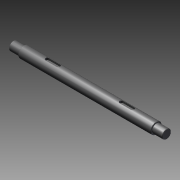
# Autodesk Inventor part: NSFRQ15-181-F14-P12-T14-Q12-WKC30-C20-K30-E20_s
Saved by Autodesk Inventor 2011 SP1 (Build 150282100, 282)
## iProperties
Created: 2016-11-24
Part Number: NSFRQ15-181-F14-P12-T14-Q12-WKC30-C20-K30-E20_s
Catalog Web Link: www.cadenas.de
Description: NSFRMHQ, SFRMHQ, PSFRMHQ, SSFRMHQ, NSFRMGQ, SFRMGQ, PSFRMGQ, SSFRMGQ, NSFRHQ, SFRHQ, PSFRHQ, SSFRHQ, NSFRQ, SFRQ, PSFRQ, SSFRQ, HFRQ, PHFRQ_shaft-Rotary Shafts - Both Ends Stepped -
Vendor: MISUMI
Document SubType Name: Modeling
Designer: psAdmin
Manufacturer: MISUMI
Mass: 34.5896 g
Surface Area: 101.193 cm^2
Volume: 34.5896 cm^3
Density: 1 g/cm^3
Category: PARTsolutions
Company: MISUMI
Title: NSFRQ15-181-F14-P12-T14-Q12-WKC30-C20-K30-E20
Author: Cadenas PARTsolutions
Comments: Rotary Shafts - Both Ends Stepped -
PSOL_IDENT_0: {$CADENAS_DATA\23d-libs\misumi\metric\11_rotary_shafts\11_components\phfrq\phfrq.prj},671 {VTYP=3D},
PSOL_IDENT_1: {NB=NSFRQ15-181-F14-P12-T14-Q12-WKC30-C20-K30-E20_s},{LINA=NSFRQ15-181-F14-P12-T14-Q12-WKC30-C20-K30
PSOL_IDENT_2: -E20},{NN=NSFRMHQ, SFRMHQ, PSFRMHQ, SSFRMHQ, NSFRMGQ, SFRMGQ, PSFRMGQ, SSFRMGQ, NSFRHQ, SFRHQ, PSFRH
PSOL_IDENT_3: Q, SSFRHQ, NSFRQ, SFRQ, PSFRQ, SSFRQ, HFRQ, PHFRQ_shaft},{DATE=20.09.2016 01:43:22},{GEOMDATE=16.09.
PSOL_IDENT_4: 2016 05:13:09},{VERSION=},{LINEID=70},{LINESUBID=-1},{WBVAR=TS,TYS,MAT,ST,ALT1,L,ALT9,F,P,T,Q,ALT2,K
PSOL_IDENT_5: C,A,WKC,C,K,E,KZ,Z,ALT8,PKC,ALT14,QKC,ALT21,PP,PK,ALT22,QQ,QK,ALT23,PV,PW,ALT24,QV,QW,ALT27,TL,TR,AL
PSOL_IDENT_6: T28,TF,ALT29,TTALT29,ALT3,FC,GALT3,WFC,J,WALT3,V,ALT4,SFC,SG,AG,ALT25,PFC,LC,ALT26,QFC,RC,ALT10,KWC,
PSOL_IDENT_7: ALT11,WC,ALT5,UC,ALT7,SC,ALT33,CPALT33,CQALT33,ALT30,PM,QM}  {NB=NSFRQ15-181-F14-P12-T14-Q12-WKC30-C
PSOL_IDENT_8: 20-K30-E20_s},{LINA=NSFRQ15-181-F14-P12-T14-Q12-WKC30-C20-K30-E20},{KT=DUMMY},{PN=NSFRQ15-181-F14-P1
PSOL_IDENT_9: 2-T14-Q12-WKC30-C20-K30-E20},{TYPE=NSFRQ},{TS=},{TYS=},{TYSALG='','g6'},{TYSS=},{TSALG='M','h9 (Cold
PSOL_IDENT_10: -drawn)','H','h7 (Ground)','','g6 (Ground)'},{MAT=S45C},{MATALG= 'S45C','S45C Equivalent', 'SUS304','
PSOL_IDENT_11: SUS304', 'SCM435','4137 Alloy Steel' },{ST=},{STALG= '','-','BO','Black Oxide', 'ENP','Electroless N
PSOL_IDENT_12: ickel Plating' },{D=15},{ALT1=},{L=181.0},{LALG=[15:796/0.1]},{LMIN=15},{LMAX=796},{LMAXLKC=799.9},{
PSOL_IDENT_13: ALT9=},{ALT9ALG= '', 'w/o CKC (Concentricity)','-CKC', 'with CKC (Concentricity)' },{F=14.0},{FALG=[
PSOL_IDENT_14: 2:70/0.1]},{FMIN=2},{FMAX=70},{P=12},{PALG=[5:14/1]},{PMIN=5},{PMIN2=0},{PMAX=14},{T=14.0},{TALG=[2:
PSOL_IDENT_15: 70/0.1]},{TMIN=2},{TMAX=70},{Q=12},{QALG=[5:14/1]},{QMIN=5},{QMIN2=0},{QMAX=14},{CIFC=0},{CC=0.5},{C
PSOL_IDENT_16: C1=0.5},{Y=800},{ALT2=WKC},{ALT2ALG= '', 'w/o Key Grooves','KC','with KC (Key Groove)','WKC','with W
PSOL_IDENT_17: KC (Two Key Grooves)','KCWKC','with KC + WKC (Three Key Grooves)','KZ','with KC + WKC + KZ (Four Key
PSOL_IDENT_18: Grooves)' },{ALT2PN=-WKC30-C20-K30-E20},{KC=0.0},{KCALG=[0]},{KCMIN=0},{KCMAX=176},{KCMAX2=166},{KC
PSOL_IDENT_19: MAX3=161},{A=0.0},{AALG=[0]},{AMIN=5},{AMAX=100},{AMAX2=100},{AMAX3=100},{WKC=30.0},{WKCALG=[0:171/0
PSOL_IDENT_20: .1]},{WKCMIN=0},{WKCMIN2=0},{WKCMAX=171},{WKCMAX2=166},{C=20.0},{CALG=[5:100/0.1]},{CMIN=5},{CMAX=10
PSOL_IDENT_21: 0},{CMAX2=100},{K=30.0},{KALG=[0:126/0.1]},{KMIN=0},{KMIN2=5},{KMAX=126},{E=20.0},{EALG=[5:100/0.1]}
PSOL_IDENT_22: ,{EMIN=5},{EMAX=100},{KZ=0.0},{KZALG=[0]},{KZMIN=151},{KZMAX=176},{Z=0.0},{ZALG=[0]},{ZMIN=5},{ZMAX=
PSOL_IDENT_23: 100},{BBALT2=5},{TTALT2=3},{ALT8=},{ALT8ALG= '','w/o PKC (Keyway on Step P (Position Zero from End F
PSOL_IDENT_24: ace))','PKC','with PKC (Keyway on Step P (Position Zero from End Face))' },{ALT8PN=},{PKC=0.0},{PKCA
PSOL_IDENT_25: LG=[0]},{PKCMIN=4},{PKCMAX=14},{ALT14=},{ALT14ALG= '','w/o QKC (Keyway on Step Q (Position Zero from
PSOL_IDENT_26: End Face))','QKC','with QKC (Keyway on Step Q (Position Zero from End Face))' },{ALT14PN=},{QKC=0.0
PSOL_IDENT_27: },{QKCALG=[0]},{QKCMIN=4},{QKCMAX=14},{ALT21=},{ALT21ALG= '','w/o PP (Keyway on Step P (Position Spe
PSOL_IDENT_28: cfied))','PP','with PP (Keyway on Step P (Position Specfied))' },{ALT21PN=},{BBALT21=2},{PP=0.0},{PP
PSOL_IDENT_29: ALG=[0]},{PPMIN1=0},{PPMIN2=0},{PPMAX=10},{PK=0.0},{PKALG=[0]},{PKMIN=4},{PKMAX=14},{ALT22=},{ALT22A
PSOL_IDENT_30: LG= '','w/o QQ (Keyway on Step Q (Position Specfied))','QQ','with QQ (Keyway on Step Q (Position Spe
PSOL_IDENT_31: cfied))' },{ALT22PN=},{QQ=0.0},{QQALG=[0]},{QQMIN1=0},{QQMIN2=0},{QQMAX=10},{QK=0.0},{QKALG=[0]},{QK
PSOL_IDENT_32: MIN=4},{QKMAX=14},{ALT23=},{ALT23ALG= '','Not applicable' },{ALT23PN=},{PV=0.0},{PVALG=[0]},{PVMIN=0
PSOL_IDENT_33: },{PVMAX=10},{PW=0.0},{PWALG=[0]},{PWMIN=4},{PWMAX=14},{ALT24=},{ALT24ALG= '','Not applicable' },{AL
PSOL_IDENT_34: T24PN=},{QV=0.0},{QVALG=[0]},{QVMIN=0},{QVMAX=10},{QW=0.0},{QWALG=[0]},{QWMIN=4},{QWMAX=14},{ALT27=}
PSOL_IDENT_35: ,{ALT27ALG= '','w/o Retaining Ring Groove at D','TL','with TL (Retaining Ring Groove at D)','TR','wi
PSOL_IDENT_36: th TR (Retaining Ring Groove at D)','TLTR','with TL + TR (Retaining Ring Groove at D)' },{ALT27PN=},
PSOL_IDENT_37: {TL=0.0},{TLALG=[0]},{TLMIN=3.2},{TLMAX=0},{TR=0.0},{TRALG=[0]},{TRMIN=3.2},{TRMAX=0},{MMALT27=1.15}
PSOL_IDENT_38: ,{DDDALT27=0},{ALT28=},{ALT28ALG= '','w/o TF (Retaining Ring Groove at Step P)','TF','with TF (Retai
PSOL_IDENT_39: ning Ring Groove at Step P)' },{ALT28PN=},{TF=0.0},{TFALG=[0]},{TFMIN=3.2},{TFMAX=12},{MMALT28ALG=1.
PSOL_IDENT_40: 15},{MMALT28=0},{DDDALT28=0},{ALT29=},{ALT29ALG= '','w/o TT (Retaining Ring Groove at Step Q)','TT','
PSOL_IDENT_41: with TT (Retaining Ring Groove at Step Q)' },{ALT29PN=},{TTALT29=0.0},{TTALT29ALG=[0]},{TTALT29MIN=3
PSOL_IDENT_42: .2},{TTALT29MAX=12},{MMALT29=0},{MMALT29ALG=1.15},{DDDALT29=0},{ALT3=},{ALT3ALG= '', 'w/o Set Screw
PSOL_IDENT_43: Flat','FC','with FC (Adds a Set Screw Flat)','WFC','with WFC (Adds Two Set Screw Flats)','FCWFC','wi
PSOL_IDENT_44: th FC + WFC (Adds Three Set Screw Flats)' },{ALT3PN=},{FC=0},{FCALG=[0]},{FCMIN=0},{FCMAX=180},{GALT
PSOL_IDENT_45: 3=0},{GALT3ALG=[0]},{GALT3MIN=1},{GALT3MAX=70},{GALT3MAX2=70},{GALT3MAX3=70},{WFC=0},{WFCALG=[0]},{W
PSOL_IDENT_46: FCMIN=0},{WFCMIN2=2},{WFCMAX=177},{WFCMAX2=-3},{WFCMAX3=-4},{J=0},{JALG=[0]},{JMIN=1},{JMAX=70},{JMA
PSOL_IDENT_47: X2=-2},{JMAX3=-5},{WALT3=0},{WALT3ALG=[0]},{WALT3MIN=0},{WALT3MIN2=183},{WALT3MAX=178},{WALT3MAX2=17
PSOL_IDENT_48: 8},{V=0},{VALG=[0]},{VMIN=1},{VMAX=70},{VMAX2=70},{CIFCUT=0},{CIFFC=0},{ALT4=},{ALT4ALG= '', 'w/o SF
PSOL_IDENT_49: C (2 Set Screw Flats (Angle Specified))', 'SFC' , 'with SFC (2 Set Screw Flats (Angle Specified))'},
PSOL_IDENT_50: {ALT4PN=},{SFC=0},{SFCALG=[0]},{SFCMIN=0},{SFCMAX=180},{SG=0},{SGALG=[0]},{SGMIN=1},{SGMAX=70},{AG=0
PSOL_IDENT_51: },{AGALG=[0]},{HALT4=0},{CIFSFC=0},{CUTSFC=0},{ALT25=},{ALT25ALG= '','w/o PFC (Set Screw Flat on Ste
PSOL_IDENT_52: p P)','PFC','with PFC (Set Screw Flat on Step P)' },{ALT25PN=},{PFC=0},{PFCALG=[0]},{PFCMN=0},{PFCMA
PSOL_IDENT_53: X=13},{LC=0},{LCALG=[0]},{LCMIN=1},{LCMAX=14},{HALT25=0},{ALT26ALG= '','w/o QFC (Set Screw Flat on S
PSOL_IDENT_54: tep Q)','QFC','with QFC (Set Screw Flat on Step Q)' },{ALT26=},{ALT26PN=},{QFC=0},{QFCALG=[0]},{QFCM
PSOL_IDENT_55: IN=0},{QFCMAX=13},{RC=0},{RCALG=[0]},{RCMIN=1},{RCMAX=14},{HALT26=0},{ALT10=},{ALT10ALG= '','w/o KWC
PSOL_IDENT_56: (2 Set Screw Flats at both ends)','KWC','with KWC (2 Set Screw Flats at both ends)' },{ALT10PN=},{K
PSOL_IDENT_57: WC=0},{KWCALG=0},{HALT10P=1.0},{HALT10Q=1.0},{ALT11=},{ALT11ALG= '','Not applicable' },{ALT11PN=},{W
PSOL_IDENT_58: C=0.0},{WCALG=0},{WCMAX=11.9},{WC1=10},{WC1MIN=9.9},{WC1MAX=10.1},{ALT5=},{ALT5ALG= '','Not applicab
PSOL_IDENT_59: le' },{ALT5PN=},{UC=0},{UCALG=[0]},{UCMIN=1},{UCMAX=175},{DD=0},{LL1=0},{ALT7=},{ALT7ALG= '', 'w/o S
PSOL_IDENT_60: C (Wrench Flats)', 'SC', 'with SC (Wrench Flats)'},{ALT7PN=},{SC=0},{SCALG=[0]},{SCMIN=0},{SCMAX=171
PSOL_IDENT_61: },{WALT7=0},{LL2=0},{LL2ALG=10},{CIFSC=0},{CUTSC=0},{TPKC=0.2},{BBALT8=4},{TTALT8=2.5},{CIFPKC=0},{T
PSOL_IDENT_62: QKC=0.2},{BBALT14=4},{TTALT14=2.5},{CIFQKC=0},{CIFR=0},{CIFR2=0},{ERRORPN=},{ERRORALT23=OK},{ERRORAL
PSOL_IDENT_63: T24=OK},{ERRORALT25=OK},{ERRORALT27=OK},{ERRORALT28=OK},{ERRORALT210=OK},{ERRORALT214=OK},{ERRORALT3
PSOL_IDENT_64: 4=OK},{ERRORALT35=OK},{ERRORALT37=OK},{ERRORALT45=OK},{ERRORALT47=OK},{ERRORALT57=OK},{CIFKG=2},{KGM
PSOL_IDENT_65: IN1=30},{KGMAX1=50},{KGMIN2=131},{KGMAX2=151},{KGMIN3=0},{KGMAX3=0},{KGMIN4=0},{KGMAX4=0},{CIFKGC=2}
PSOL_IDENT_66: ,{CIFKG1=0},{CIFKG2=0},{CIFKG3=0},{CIFKG4=0},{CIFKGPCUT=0},{CIFKGQCUT=0},{PCUT3D=0},{QCUT3D=0},{CIFK
PSOL_IDENT_67: GP=0},{KGPMIN1=0},{KGPMAX1=0},{KGPMIN2=0},{KGPMAX2=0},{KGPMIN3=0},{KGPMAX3=0},{CIFKGPC=0},{CIFKGP1=1
PSOL_IDENT_68: },{CIFKGQ=0},{KGQMIN1=0},{KGQMAX1=0},{KGQMIN2=0},{KGQMAX2=0},{KGQMIN3=0},{KGQMAX3=0},{CIFKGQC=0},{CI
PSOL_IDENT_69: FKGQ1=1},{ALT33=},{ALT33ALG= '', 'w/o Step Chamfering','CP','with CP (Step P Chamfering)','CQ','with
PSOL_IDENT_70: CQ (Step Q Chamfering)','CPCQ','with CP + CQ (Step Chamfering at Both Steps)' },{ALT33PN=},{CPALT33=
PSOL_IDENT_71: },{CPALT33ALG= '','N/A' },{CPALT333D=0.5},{CQALT33=},{CQALT33ALG= '','N/A' },{CQALT333D=0.5},{CIF33P
PSOL_IDENT_72: FC=0},{CIF33QFC=0},{CIF33KWCP=0},{CIF33KWCQ=0},{CIF33TFP=0},{CIF33TTQ=0},{ERRORALT221=OK},{ERRORALT2
PSOL_IDENT_73: 22=OK},{ERRORALT223=OK},{ERRORALT224=OK},{ERRORALT225=OK},{ERRORALT226=OK},{ERRORALT227=OK},{ERRORAL
PSOL_IDENT_74: T228=OK},{ERRORALT229=OK},{ERRORALT230=OK},{ERRORALT310=OK},{ERRORALT327=OK},{ERRORALT330=OK},{ERROR
PSOL_IDENT_75: ALT410=OK},{ERRORALT427=OK},{ERRORALT430=OK},{ERRORALT510=OK},{ERRORALT527=OK},{ERRORALT530=OK},{ERR
PSOL_IDENT_76: ORALT710=OK},{ERRORALT730=OK},{ERRORALT825=OK},{ERRORALT828=OK},{ERRORALT830=OK},{ERRORALT1030=OK},{
PSOL_IDENT_77: ERRORALT1426=OK},{ERRORALT1429=OK},{ERRORALT1430=OK},{ERRORALT2125=OK},{ERRORALT2128=OK},{ERRORALT21
PSOL_IDENT_78: 30=OK},{ERRORALT2226=OK},{ERRORALT2229=OK},{ERRORALT2230=OK},{ERRORALT2325=OK},{ERRORALT2328=OK},{ER
PSOL_IDENT_79: RORALT2426=OK},{ERRORALT2429=OK},{ERRORALT2528=OK},{ERRORALT2530=OK},{ERRORALT2629=OK},{ERRORALT2630=
PSOL_IDENT_80: OK},{ERRORALT2830=OK},{ERRORALT2930=OK},{ALT30=},{ALT30ALG= '','w/o Tapping','PM','with PM (Tapping)'
PSOL_IDENT_81: ,'QM','with QM (Tapping)','PMQM','with PM + QM (Tapping)' },{ALT30PN=},{PM=0},{PMALG= 0 },{QM=0},{QM
PSOL_IDENT_82: ALG=0},{PM3D=0},{QM3D=0},{CIFPM=0},{CIFQM=0},{PMPITCH=0},{QMPITCH=0},{PMDEEP=0},{QMDEEP=0},{CIFCALC1=
PSOL_IDENT_83: 20},{CIFCALC2=20},{CIFCALC3=0},{CIFCALC4=0},{CIFPCALC1=0},{CIFPCALC2=0},{CIFPCALC3=0},{CIFQCALC1=0},
PSOL_IDENT_84: {CIFQCALC2=0},{CIFQCALC3=0},{QMALG1=0},{QMALG2=0}
NN: NSFRMHQ, SFRMHQ, PSFRMHQ, SSFRMHQ, NSFRMGQ, SFRMGQ, PSFRMGQ, SSFRMGQ, NSFRHQ, SFRHQ, PSFRHQ, SSFRHQ, NSFRQ, SFRQ, PSFRQ, SSFRQ, HFRQ, PHFRQ_shaft
NT: Rotary Shafts - Both Ends Stepped -
NB: NSFRQ15-181-F14-P12-T14-Q12-WKC30-C20-K30-E20_s
NBSYN: $PN._s
LINA: NSFRQ15-181-F14-P12-T14-Q12-WKC30-C20-K30-E20
PN: NSFRQ15-181-F14-P12-T14-Q12-WKC30-C20-K30-E20
TS: g6 (Ground)
TYS: g6
MAT: S45C Equivalent
ST: -
D: 15
ALT1: w/o LKC (Changes L Tolerance)
L: 181.0
ALT9: w/o CKC (Concentricity)
F: 14.0
P: 12
T: 14.0
Q: 12
Y: 800
ALT2: with WKC (Two Key Grooves)
KC: 0.0
A: 0.0
WKC: 30.0
C: 20.0
K: 30.0
E: 20.0
KZ: 0.0
Z: 0.0
ALT8: w/o PKC (Keyway on Step P (Position Zero from End Face))
PKC: 0.0
ALT14: w/o QKC (Keyway on Step Q (Position Zero from End Face))
QKC: 0.0
ALT21: w/o PP (Keyway on Step P (Position Specfied))
PP: 0.0
PK: 0.0
ALT22: w/o QQ (Keyway on Step Q (Position Specfied))
QQ: 0.0
QK: 0.0
ALT23: Not applicable
PV: 0.0
PW: 0.0
ALT24: Not applicable
QV: 0.0
QW: 0.0
ALT27: w/o Retaining Ring Groove at D
TL: 0.0
TR: 0.0
ALT28: w/o TF (Retaining Ring Groove at Step P)
TF: 0.0
ALT29: w/o TT (Retaining Ring Groove at Step Q)
TTALT29: 0.0
ALT3: w/o Set Screw Flat
FC: 0
GALT3: 0
WFC: 0
J: 0
WALT3: 0
V: 0
ALT4: w/o SFC (2 Set Screw Flats (Angle Specified))
SFC: 0
SG: 0
AG: 0
HALT4: 0
ALT25: w/o PFC (Set Screw Flat on Step P)
PFC: 0
LC: 0
ALT26: w/o QFC (Set Screw Flat on Step Q)
QFC: 0
RC: 0
ALT10: w/o KWC (2 Set Screw Flats at both ends)
KWC: 0
ALT11: Not applicable
WC: 0.0
ALT5: Not applicable
UC: 0
DD: 0
LL1: 0
ALT7: w/o SC (Wrench Flats)
SC: 0
WALT7: 0
LL2: 0
ALT33: w/o Step Chamfering
CPALT33: N/A
CQALT33: N/A
ALT30: w/o Tapping
PM: 0
QM: 0
SUPPLIER: MISUMI
ARTICLENO: NSFRQ15-181-F14-P12-T14-Q12-WKC30-C20-K30-E20_s
BOMINFO: NSFRQ15-181-F14-P12-T14-Q12-WKC30-C20-K30-E20
CREATOR: CADENAS GmbH
Autodesk Inventor part; units mm, degrees
ref_plane "YZ Plane" through (0, 0, 0) normal (1, 0, 0) x (0, 1, 0)
ref_plane "XZ Plane" through (0, 0, 0) normal (0, 1, 0) x (-1, 0, 0)
ref_plane "XY Plane" through (0, 0, 0) normal (0, 0, 1) x (1, 0, 0)
sketch "Sketch_1" plane through (0, 0, 0) normal (0, 0, 1) x (1, 0, 0)
  line L0 (195, 0) -> (-14, 0)
  line L1 (-14, 0) -> (-14, 5.5)
  line L2 (-14, 5.5) -> (-13.5, 6)
  line L3 (-13.5, 6) -> (-0.2, 6)
  arc A0 (-0.2, 6) -> (0, 6.2) centre (-0.2, 6.2) ccw
  line L4 (0, 6.2) -> (0, 7)
  line L5 (0, 7) -> (0.5, 7.5)
  line L6 (0.5, 7.5) -> (180.5, 7.5)
  line L7 (180.5, 7.5) -> (181, 7)
  line L8 (181, 7) -> (181, 6.2)
  arc A1 (181, 6.2) -> (181.2, 6) centre (181.2, 6.2) ccw
  line L9 (181.2, 6) -> (194.5, 6)
  line L10 (194.5, 6) -> (195, 5.5)
  line L11 (195, 5.5) -> (195, 0)
  line L12 (195, 0) -> (-14, 0)
  constraints: 26 end point, 4 point on circle, 2 centre point
revolve "Revolution1" add sketch "Sketch_1" angle 360 about axis through (195, 0, 0) along (1, 0, 0)
sketch "_____2" plane through (0, 0, 7.5) normal (0, 0, 1) x (1, 0, 0)
  arc A0 (32.5, 2.5) -> (32.5, -2.5) centre (32.5, 0) ccw
  line L0 (32.5, -2.5) -> (47.5, -2.5)
  arc A1 (47.5, -2.5) -> (47.5, 2.5) centre (47.5, 0) ccw
  line L1 (47.5, 2.5) -> (32.5, 2.5)
  constraints: 4 end point, 4 point on circle, 2 centre point
extrude "Extrusion1" cut sketch "_____2" against normal blind 3
sketch "_____6" plane through (0, 0, 7.5) normal (0, 0, 1) x (1, 0, 0)
  arc A0 (133.5, 2.5) -> (133.5, -2.5) centre (133.5, 0) ccw
  line L0 (133.5, -2.5) -> (148.5, -2.5)
  arc A1 (148.5, -2.5) -> (148.5, 2.5) centre (148.5, 0) ccw
  line L1 (148.5, 2.5) -> (133.5, 2.5)
  constraints: 4 end point, 4 point on circle, 2 centre point
extrude "Extrusion2" cut sketch "_____6" against normal blind 3
body "Solid1"
